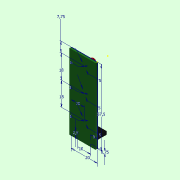
# Autodesk Inventor part: Led_Board_V1
Saved by Autodesk Inventor 2015 (Build 190159000, 159)
## iProperties
Created: 2014-12-24
Part Number: Led_Board_V1
Material: Generic
Document SubType Name: Modeling
Designer: Openlab
Density: 1 g/cm^3
Appearance: Smooth - Dark Forest Green
Mass: 2.60407 g
Surface Area: 31.9711 cm^2
Volume: 2.60407 cm^3
Author: Openlab
Autodesk Inventor part; units mm, degrees
ref_plane "YZ Plane" through (0, 0, 0) normal (1, 0, 0) x (0, 1, 0)
ref_plane "XZ Plane" through (0, 0, 0) normal (0, 1, 0) x (-1, 0, 0)
ref_plane "XY Plane" through (0, 0, 0) normal (0, 0, 1) x (1, 0, 0)
sketch "Sketch1" plane through (0, 0, 0) normal (0, 1, 0) x (-1, 0, 0)
  line L0 (20, 0) -> (0, 0)
  line L1 (0, 0) -> (0, -57.5)
  line L2 (0, -57.5) -> (20, -57.5)
  line L3 (20, -57.5) -> (20, 0)
  circle A0 centre (10, -7.75) radius 2.5
  circle A1 centre (10, -25.75) radius 2.5
  circle A2 centre (10, -43.75) radius 2.5
  line L4 (15, -54.25) -> (5, -54.25)
  line L5 (5, -54.25) -> (5, -56.75)
  line L6 (5, -56.75) -> (15, -56.75)
  line L7 (15, -56.75) -> (15, -54.25)
  circle A3 centre (10, -7.75) radius 3
  circle A4 centre (10, -25.75) radius 3
  circle A5 centre (10, -43.75) radius 3
  dimension "d0" = 57.5
  dimension "d1" = 20
  dimension "d2" = 5
  dimension "d3" = 5
  dimension "d4" = 5
  dimension "d8" = 0.75
  dimension "d9" = 2.5
  dimension "d10" = 10
  dimension "d20" = 10
  dimension "d21" = 5
  dimension "d22" = 6
  dimension "d23" = 6
  dimension "d24" = 6
  dimension "d45" = 7.75
  dimension "d46" = 18
  dimension "d47" = 18
  constraints: 16 end point, 6 centre point, 4 coincident, 4 parallel, 2 horizontal, 2 perpendicular, 2 vertical alignment
  measures "d0" distance of L0.end L1.end
  measures "d1" distance of L1.end L2.end
  measures "d2" diameter of A0
  measures "d3" diameter of A1
  measures "d4" diameter of A2
  measures "d8" distance between parallel lines of L2 L6
  measures "d9" distance of L6.end L4.start
  measures "d10" distance of L5.end L6.end
  measures "d20" distance from line of L3 A2.centre
  measures "d21" distance between parallel lines of L1 L5
  measures "d22" diameter of A3
  measures "d23" diameter of A4
  measures "d24" diameter of A5
  measures "d45" distance from line of L0 A0.centre
  measures "d46" distance of A1.centre A0.centre
  measures "d47" distance of A2.centre A1.centre
extrude "Extrusion1" add sketch "Sketch1" against normal blind 1.4 contours L3 L2 L1 L0 | A0 | A1 | A2 | L7 L6 L5 L4 | A3 | A4 | A5
extrude "Extrusion2" add sketch "Sketch1" along normal blind 12 contours L7 L6 L5 L4
extrude "Extrusion5" add sketch "Sketch1" along normal blind 8 contours A0
extrude "Extrusion6" add sketch "Sketch1" along normal blind 1 contours A3
fillet "Fillet4" radius 2.5 1 edges at (-7.5, 8, -7.75)
extrude "Extrusion7" add sketch "Sketch1" along normal blind 1 contours A4
extrude "Extrusion8" add sketch "Sketch1" along normal blind 8 contours A1
fillet "Fillet5" [suppressed]
extrude "Extrusion9" add sketch "Sketch1" along normal blind 8 contours A2
extrude "Extrusion10" add sketch "Sketch1" along normal blind 1 contours A5
fillet "Fillet6" radius 2.5 1 edges at (-7.5, 8, -43.75)
sketch "Sketch2" plane through (-10, 8, -25.75) normal (0, 1, 0) x (1, 0, 0)
  point P0 (10, -25.75)
  point P1 (0, 0)
body "Solid1"
